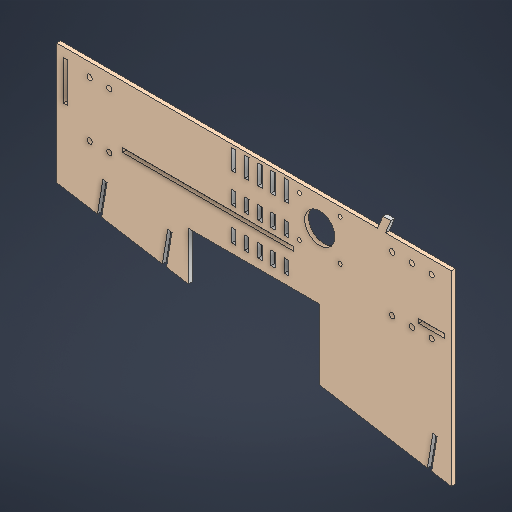
# Autodesk Inventor part: Sideboard
Saved by Autodesk Inventor 2027 (Build 310192000, 192)
## iProperties
Created: 2026-05-09
Part Number: Sideboard
Material: Generic
Document SubType Name: Modeling
Designer: alexy
Density: 1 g/cm^3
Appearance: Default
Author: alexy
Autodesk Inventor part; units mm, degrees
ref_plane "YZ Plane" through (0, 0, 0) normal (1, 0, 0) x (0, 1, 0)
ref_plane "XZ Plane" through (0, 0, 0) normal (0, 1, 0) x (-1, 0, 0)
ref_plane "XY Plane" through (0, 0, 0) normal (0, 0, 1) x (1, 0, 0)
sketch "Sketch1" plane through (0, 0, 0) normal (0, 0, 1) x (1, 0, 0)
  line L0 (0, 0) -> (300, 0)
  line L1 (300, 0) -> (300, 62)
  line L2 (300, 62) -> (0, 62)
  line L3 (0, 62) -> (0, 0)
  circle A0 centre (184.5, 55.5) radius 1.55
  circle A1 centre (184.5, 24.5) radius 1.55
  circle A2 centre (215.5, 55.5) radius 1.55
  circle A3 centre (215.5, 24.5) radius 1.55
  circle A4 centre (200, 40) radius 11.5
  line L4 (50, 18.1) -> (180, 18.1)
  line L5 (180, 18.1) -> (180, 15)
  line L6 (180, 15) -> (50, 15)
  line L7 (50, 15) -> (50, 18.1)
  line L8 (0, 62) -> (39.6145, 62)
  line L9 (8.1, 25) -> (5, 25)
  line L10 (5, 25) -> (5, 55)
  line L11 (5, 55) -> (8.1, 55)
  line L12 (8.1, 55) -> (8.1, 25)
  line L13 (8.1, 25) -> (5, 55) construction
  line L14 (5, 25) -> (8.1, 55) construction
  circle A5 centre (285, 10) radius 2.05
  circle A6 centre (270, 10) radius 2.05
  circle A7 centre (285, 52) radius 2.05
  circle A8 centre (270, 52) radius 2.05
  circle A9 centre (255, 52) radius 2.05
  circle A10 centre (255, 10) radius 2.05
  circle A11 centre (40, 10) radius 2.05
  circle A12 centre (25, 10) radius 2.05
  circle A13 centre (40, 52) radius 2.05
  circle A14 centre (25, 52) radius 2.05
  line L15 (275, 18.1) -> (295, 18.1)
  line L16 (295, 18.1) -> (295, 15)
  line L17 (295, 15) -> (275, 15)
  line L18 (275, 15) -> (275, 18.1)
  line L19 (0, 62) -> (50, 62)
  point P0 (6.55, 40)
  point P1 (5, 40)
  point P2 (8.1, 40)
  point P3 (50, 16.55)
  point P4 (180, 16.55)
  dimension "d1" = 3.1
  dimension "d2" = 3.1
  dimension "d3" = 3.1
  dimension "d4" = 3.1
  dimension "d5" = 31
  dimension "d7" = 23
  dimension "d8" = 15.5
  dimension "d9" = 15.5
  dimension "d10" = 62
  dimension "d11" = 31
  dimension "d12" = 3.1
  dimension "d13" = 40
  dimension "d54" = 300
  dimension "d55" = 3.1
  dimension "d56" = 5
  dimension "d57" = 15
  dimension "d59" = 130
  dimension "d63" = 4.1
  dimension "d64" = 4.1
  dimension "d65" = 4.1
  dimension "d66" = 4.1
  dimension "d67" = 4.1
  dimension "d68" = 4.1
  dimension "d69" = 15
  dimension "d70" = 15
  dimension "d71" = 10
  dimension "d72" = 10
  dimension "d73" = 15
  dimension "d79" = 4.1
  dimension "d80" = 4.1
  dimension "d81" = 4.1
  dimension "d82" = 4.1
  dimension "d85" = 15
  dimension "d87" = 10
  dimension "d88" = 10
  dimension "d89" = 10
  dimension "d91" = 5
  dimension "d92" = 20
  dimension "d93" = 15
  dimension "d106" = 20
  dimension "d107" = 50
  constraints: 40 end point, 15 centre point, 11 horizontal alignment, 8 parallel, 7 vertical alignment, 6 midpoint, 5 horizontal, 4 perpendicular
  measures "d1" diameter of A0
  measures "d2" diameter of A1
  measures "d3" diameter of A2
  measures "d4" diameter of A3
  measures "d5" distance of A1.centre A3.centre
  measures "d7" diameter of A4
  measures "d8" horizontal distance of A0.centre A4.centre
  measures "d9" horizontal distance of A4.centre A3.centre
  measures "d10" distance of L0.end L1.end
  measures "d11" distance of A3.centre A2.centre
  measures "d12" distance of L6.end L4.start
  measures "d13" distance from line of L0 A4.centre
  measures "d54" distance of L0.end L0.start
  measures "d55" distance of L10.end L11.end
  measures "d56" distance between parallel lines of L3 L10
  measures "d57" distance of point (5, 40) L10.end
  measures "d59" distance of L5.end L6.end
  measures "d63" diameter of A5
  measures "d64" diameter of A6
  measures "d65" diameter of A7
  measures "d66" diameter of A8
  measures "d67" diameter of A9
  measures "d68" diameter of A10
  measures "d69" distance of A6.centre A5.centre
  measures "d70" distance of A10.centre A6.centre
  measures "d71" distance from line of L0 A5.centre
  measures "d72" distance from line of L2 A7.centre
  measures "d73" distance from line of L1 A5.centre
  measures "d79" diameter of A11
  measures "d80" diameter of A12
  measures "d81" diameter of A13
  measures "d82" diameter of A14
  measures "d85" distance of A12.centre A11.centre
  measures "d87" horizontal distance of A11.centre L6.end
  measures "d88" distance from line of L0 A11.centre
  measures "d89" distance from line of L2 A13.centre
  measures "d91" distance between parallel lines of L1 L16
  measures "d92" distance between parallel lines of L16 L18
  measures "d93" distance between parallel lines of L0 L6
  measures "d106" horizontal distance of point (180, 16.55) A4.centre
  measures "d107" distance from line of L3 point (50, 16.55)
extrude "Extrusion1" add sketch "Sketch1" along normal blind 3
sketch "Sketch4" plane through (0, 0, 3) normal (0, 0, 1) x (1, 0, 0)
  line L0 (300, 62) -> (0, 62) projected
  line L1 (244, 62) -> (248, 72)
  line L2 (248, 72) -> (254, 72)
  line L3 (254, 72) -> (250, 62)
  point P0 (0, 0)
  dimension "d108" = 10
  dimension "d109" = 4
  dimension "d110" = 50
  dimension "d111" = 6
  constraints: 6 end point, 2 parallel, 2 point on line
  measures "d108" distance from line of L0 L1.end
  measures "d109" horizontal distance of L1.start L1.end
  measures "d110" distance of L0.start L3.end
  measures "d111" distance of L2.end L1.end
extrude "Extrusion4" add sketch "Sketch4" against normal blind 3
sketch "Sketch5" plane through (0, 0, 3) normal (0, 0, 1) x (1, 0, 0)
  line L0 (0, 0) -> (300, 0) projected
  line L1 (0, -30) -> (300, -80)
  line L2 (300, -80) -> (300, 0)
  line L3 (100, -46.6667) -> (100, 0)
  line L4 (200, -63.3333) -> (200, 0)
  line L5 (0, 0) -> (0, -30)
  line L6 (80.2721, -43.3787) -> (84.415, -18.5216)
  line L7 (84.415, -18.5216) -> (87.5714, -19.0476)
  line L8 (87.5714, -19.0476) -> (83.4286, -43.9048)
  line L9 (80.2721, -43.3787) -> (83.4286, -43.9048)
  line L10 (35.0953, -10.3016) -> (38.2517, -10.8277)
  line L11 (38.2517, -10.8277) -> (34.1089, -35.6848)
  line L12 (30.9524, -35.1587) -> (35.0953, -10.3016)
  line L13 (30.9524, -35.1587) -> (34.1089, -35.6848)
  line L14 (100, -10) -> (200, -10)
  line L15 (285, -77.5) -> (289.1429, -52.6429)
  line L16 (289.1429, -52.6429) -> (285.9864, -52.1168)
  line L17 (285.9864, -52.1168) -> (281.8435, -76.9739)
  point P0 (-183.9333, 0)
  dimension "d114" = 100
  dimension "d115" = 100
  dimension "d116" = 80
  dimension "d137" = 30
  dimension "d138" = 25.2
  dimension "d139" = 3.2
  dimension "d141" = 20
  dimension "d142" = 25.2
  dimension "d143" = 3.2
  dimension "d146" = 50
  dimension "d175" = 10
  dimension "d196" = 0
  dimension "d198" = 25.2
  dimension "d199" = 3.2
  dimension "d200" = 15
  constraints: 34 end point, 10 perpendicular, 10 point on line, 1 parallel, 1 vertical
  measures "d114" distance between parallel lines of L2 L4
  measures "d115" distance from line of L0.start L3
  measures "d116" distance of L0.end L1.end
  measures "d137" distance of L0.start L1.start
  measures "d138" distance between parallel lines of L9 L7
  measures "d139" distance between parallel lines of L6 L8
  measures "d141" distance from line of L3.start L6
  measures "d142" distance between parallel lines of L13 L10
  measures "d143" distance between parallel lines of L12 L11
  measures "d146" distance between parallel lines of L8 L11
  measures "d175" distance between parallel lines of L0 L14
  measures "d196" distance between parallel lines of L1 L13
  measures "d198" distance of L15.start L15.end
  measures "d199" distance of L15.end L16.end
  measures "d200" horizontal distance of L1.end L15.start
extrude "Extrusion5" add sketch "Sketch5" against normal blind 3 contours L0 L3 L1 L8 L7 L6 L11 L10 L12 L5 | L0 L4 L14 L3 | L0 L2 L1 L15 L16 L17 L4
sketch "Sketch7" plane through (0, 0, 3) normal (0, 0, 1) x (1, 0, 0)
  line L0 (172.9, 59.6) -> (176.1, 59.6)
  line L1 (176.1, 59.6) -> (176.1, 44.4)
  line L2 (176.1, 44.4) -> (172.9, 44.4)
  line L3 (172.9, 44.4) -> (172.9, 59.6)
  line L4 (172.9, 59.6) -> (176.1, 44.4) construction
  line L5 (176.1, 59.6) -> (172.9, 44.4) construction
  line L6 (172.9, 32.1) -> (176.1, 32.1)
  line L7 (176.1, 32.1) -> (176.1, 21.9)
  line L8 (176.1, 21.9) -> (172.9, 21.9)
  line L9 (172.9, 21.9) -> (172.9, 32.1)
  line L10 (172.9, 32.1) -> (176.1, 21.9) construction
  line L11 (176.1, 32.1) -> (172.9, 21.9) construction
  line L12 (244, 62) -> (0, 62) projected
  circle A0 centre (184.5, 55.5) radius 1.55 projected
  line L13 (162.9, 59.6) -> (166.1, 59.6)
  line L14 (166.1, 59.6) -> (166.1, 44.4)
  line L15 (166.1, 44.4) -> (162.9, 44.4)
  line L16 (162.9, 44.4) -> (162.9, 59.6)
  line L17 (162.9, 59.6) -> (166.1, 44.4) construction
  line L18 (166.1, 59.6) -> (162.9, 44.4) construction
  line L19 (162.9, 32.1) -> (166.1, 32.1)
  line L20 (166.1, 32.1) -> (166.1, 21.9)
  line L21 (166.1, 21.9) -> (162.9, 21.9)
  line L22 (162.9, 21.9) -> (162.9, 32.1)
  line L23 (162.9, 32.1) -> (166.1, 21.9) construction
  line L24 (166.1, 32.1) -> (162.9, 21.9) construction
  line L25 (152.9, 59.6) -> (156.1, 59.6)
  line L26 (156.1, 59.6) -> (156.1, 44.4)
  line L27 (156.1, 44.4) -> (152.9, 44.4)
  line L28 (152.9, 44.4) -> (152.9, 59.6)
  line L29 (152.9, 59.6) -> (156.1, 44.4) construction
  line L30 (156.1, 59.6) -> (152.9, 44.4) construction
  line L31 (152.9, 32.1) -> (156.1, 32.1)
  line L32 (156.1, 32.1) -> (156.1, 21.9)
  line L33 (156.1, 21.9) -> (152.9, 21.9)
  line L34 (152.9, 21.9) -> (152.9, 32.1)
  line L35 (152.9, 32.1) -> (156.1, 21.9) construction
  line L36 (156.1, 32.1) -> (152.9, 21.9) construction
  line L37 (142.9, 59.6) -> (146.1, 59.6)
  line L38 (146.1, 59.6) -> (146.1, 44.4)
  line L39 (146.1, 44.4) -> (142.9, 44.4)
  line L40 (142.9, 44.4) -> (142.9, 59.6)
  line L41 (142.9, 59.6) -> (146.1, 44.4) construction
  line L42 (146.1, 59.6) -> (142.9, 44.4) construction
  line L43 (142.9, 32.1) -> (146.1, 32.1)
  line L44 (146.1, 32.1) -> (146.1, 21.9)
  line L45 (146.1, 21.9) -> (142.9, 21.9)
  line L46 (142.9, 21.9) -> (142.9, 32.1)
  line L47 (142.9, 32.1) -> (146.1, 21.9) construction
  line L48 (146.1, 32.1) -> (142.9, 21.9) construction
  line L49 (132.9, 59.6) -> (136.1, 59.6)
  line L50 (136.1, 59.6) -> (136.1, 44.4)
  line L51 (136.1, 44.4) -> (132.9, 44.4)
  line L52 (132.9, 44.4) -> (132.9, 59.6)
  line L53 (132.9, 59.6) -> (136.1, 44.4) construction
  line L54 (136.1, 59.6) -> (132.9, 44.4) construction
  line L55 (132.9, 32.1) -> (136.1, 32.1)
  line L56 (136.1, 32.1) -> (136.1, 21.9)
  line L57 (136.1, 21.9) -> (132.9, 21.9)
  line L58 (132.9, 21.9) -> (132.9, 32.1)
  line L59 (132.9, 32.1) -> (136.1, 21.9) construction
  line L60 (136.1, 32.1) -> (132.9, 21.9) construction
  line L61 (172.9, 7.1) -> (176.1, 7.1)
  line L62 (176.1, 7.1) -> (176.1, -3.1)
  line L63 (176.1, -3.1) -> (172.9, -3.1)
  line L64 (172.9, -3.1) -> (172.9, 7.1)
  line L65 (172.9, 7.1) -> (176.1, -3.1) construction
  line L66 (176.1, 7.1) -> (172.9, -3.1) construction
  line L67 (166.1, 7.1) -> (166.1, -3.1)
  line L68 (166.1, -3.1) -> (162.9, -3.1)
  line L69 (162.9, 7.1) -> (166.1, 7.1)
  line L70 (162.9, -3.1) -> (162.9, 7.1)
  line L71 (162.9, 7.1) -> (166.1, -3.1) construction
  line L72 (166.1, 7.1) -> (162.9, -3.1) construction
  line L73 (156.1, 7.1) -> (156.1, -3.1)
  line L74 (156.1, -3.1) -> (152.9, -3.1)
  line L75 (152.9, 7.1) -> (156.1, 7.1)
  line L76 (152.9, -3.1) -> (152.9, 7.1)
  line L77 (152.9, 7.1) -> (156.1, -3.1) construction
  line L78 (156.1, 7.1) -> (152.9, -3.1) construction
  line L79 (146.1, 7.1) -> (146.1, -3.1)
  line L80 (146.1, -3.1) -> (142.9, -3.1)
  line L81 (142.9, 7.1) -> (146.1, 7.1)
  line L82 (142.9, -3.1) -> (142.9, 7.1)
  line L83 (142.9, 7.1) -> (146.1, -3.1) construction
  line L84 (146.1, 7.1) -> (142.9, -3.1) construction
  line L85 (136.1, 7.1) -> (136.1, -3.1)
  line L86 (136.1, -3.1) -> (132.9, -3.1)
  line L87 (132.9, 7.1) -> (136.1, 7.1)
  line L88 (132.9, -3.1) -> (132.9, 7.1)
  line L89 (132.9, 7.1) -> (136.1, -3.1) construction
  line L90 (136.1, 7.1) -> (132.9, -3.1) construction
  point P0 (0, 0)
  point P1 (174.5, 52)
  point P2 (174.5, 27)
  point P3 (164.5, 52)
  point P4 (164.5, 27)
  point P5 (154.5, 52)
  point P6 (154.5, 27)
  point P7 (144.5, 52)
  point P8 (144.5, 27)
  point P9 (134.5, 52)
  point P10 (134.5, 27)
  point P11 (172.9, 52)
  point P12 (152.9, 52)
  point P13 (174.5, 2)
  point P14 (164.5, 2)
  point P15 (154.5, 2)
  point P16 (144.5, 2)
  point P17 (134.5, 2)
  point P18 (172.9, 2)
  point P19 (152.9, 2)
  dimension "d147" = 3.2
  dimension "d148" = 15.2
  dimension "d149" = 10.2
  dimension "d150" = 25
  dimension "d151" = 10
  dimension "d152" = 10
  dimension "d153" = 3.2
  dimension "d154" = 15.2
  dimension "d155" = 10.2
  dimension "d156" = 25
  dimension "d157" = 3.2
  dimension "d158" = 15.2
  dimension "d159" = 10.2
  dimension "d160" = 25
  dimension "d161" = 3.2
  dimension "d162" = 15.2
  dimension "d163" = 10.2
  dimension "d164" = 25
  dimension "d165" = 3.2
  dimension "d166" = 15.2
  dimension "d167" = 10.2
  dimension "d168" = 25
  dimension "d169" = 10
  dimension "d170" = 10
  dimension "d171" = 10
  dimension "d172" = 10
  dimension "d181" = 3.2
  dimension "d182" = 10.2
  dimension "d183" = 3.2
  dimension "d184" = 10.2
  dimension "d185" = 3.2
  dimension "d186" = 10.2
  dimension "d187" = 3.2
  dimension "d188" = 10.2
  dimension "d189" = 3.2
  dimension "d190" = 10.2
  dimension "d191" = 10
  dimension "d192" = 10
  dimension "d193" = 10
  dimension "d194" = 10
  dimension "d195" = 25
  constraints: 180 end point, 34 midpoint, 30 parallel, 15 horizontal, 15 perpendicular, 8 horizontal alignment, 6 vertical alignment, 5 point on line
  measures "d147" distance of L1.end L2.end
  measures "d148" distance of L2.end L0.start
  measures "d149" distance of L8.end L6.start
  measures "d150" distance of point (174.5, 27) point (174.5, 52)
  measures "d151" distance from line of L12 point (174.5, 52)
  measures "d152" horizontal distance of A0.centre point (174.5, 52)
  measures "d153" distance of L14.end L15.end
  measures "d154" distance of L15.end L13.start
  measures "d155" distance of L22.start L19.start
  measures "d156" distance of point (164.5, 27) point (164.5, 52)
  measures "d157" distance of L26.end L27.end
  measures "d158" distance of L27.end L25.start
  measures "d159" distance of L34.start L31.start
  measures "d160" distance of point (154.5, 27) point (154.5, 52)
  measures "d161" distance of L38.end L39.end
  measures "d162" distance of L39.end L37.start
  measures "d163" distance of L46.start L43.start
  measures "d164" distance of point (144.5, 27) point (144.5, 52)
  measures "d165" distance of L50.end L51.end
  measures "d166" distance of L51.end L49.start
  measures "d167" distance of L58.start L55.start
  measures "d168" distance of point (134.5, 27) point (134.5, 52)
  measures "d169" distance of point (164.5, 52) point (174.5, 52)
  measures "d170" distance of point (164.5, 52) point (154.5, 52)
  measures "d171" distance of point (144.5, 52) point (154.5, 52)
  measures "d172" distance of point (134.5, 52) point (144.5, 52)
  measures "d181" distance of L63.start L63.end
  measures "d182" distance of L63.end L64.end
  measures "d183" distance of L67.end L70.start
  measures "d184" distance of L70.start L70.end
  measures "d185" distance of L73.end L78.end
  measures "d186" distance of L78.end L75.start
  measures "d187" distance of L79.end L82.start
  measures "d188" distance of L82.start L82.end
  measures "d189" distance of L85.end L86.end
  measures "d190" distance of L86.end L89.start
  measures "d191" distance of point (164.5, 2) point (174.5, 2)
  measures "d192" distance of point (164.5, 2) point (154.5, 2)
  measures "d193" distance of point (144.5, 2) point (154.5, 2)
  measures "d194" distance of point (134.5, 2) point (144.5, 2)
  measures "d195" distance of point (174.5, 2) point (174.5, 27)
extrude "Extrusion6" cut sketch "Sketch7" against normal blind 3 contours L0 L1 L2 L3 | L6 L7 L8 L9 | L13 L14 L15 L16 | L19 L20 L21 L22 | L25 L26 L27 L28 | L31 L32 L33 L34 | L37 L38 L39 L40 | L43 L44 L45 L46 | L49 L50 L51 L52 | L55 L56 L57 L58 | L61 L62 L63 L64 | L67 L68 L70 L69 | L73 L74 L76 L75 | L79 L80 L82 L81 | L85 L86 L88 L87
body "Solid1"
